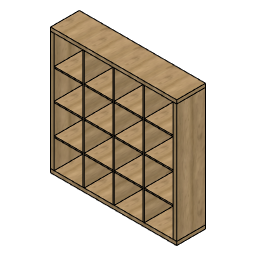
Kast+parametrisch+v5 (Autodesk Fusion 360 design; units mm, degrees)
part number: 123
Autodesk Fusion 360 part; units mm, degrees
sketch "Sketch1" plane through (0, 0, 0) normal (0, 0, 1) x (1, 0, 0)
  line L0 (0, 0) -> (50, 0)
  line L1 (50, 0) -> (50, 1654)
  line L2 (50, 1654) -> (0, 1654)
  line L3 (0, 1654) -> (0, 0)
  line L4 (0, 0) -> (1754, 0)
  line L5 (1754, 0) -> (1754, -50)
  line L6 (1754, -50) -> (0, -50)
  line L7 (0, -50) -> (0, 0)
  line L8 (450, 0) -> (468, 0)
  line L9 (468, 0) -> (468, 1654)
  line L10 (468, 1654) -> (450, 1654)
  line L11 (450, 1654) -> (450, 0)
  line L12 (50, 400) -> (450, 400)
  line L13 (450, 400) -> (450, 418)
  line L14 (450, 418) -> (50, 418)
  line L15 (50, 418) -> (50, 400)
  dimension "d7" = 1654
  dimension "d8" = 50
  dimension "d9" = 1754
  dimension "d10" = 50
  dimension "d12" = 18
  dimension "d13" = 400
  dimension "d14" = 1654
  dimension "d15" = 18
  dimension "d16" = 400
  constraint horizontal L0
  constraint vertical L1
  constraint horizontal L2
  constraint vertical L3
  constraint coincident L0.start L3.end
  constraint horizontal L4
  constraint vertical L5
  constraint horizontal L6
  constraint vertical L7
  constraint horizontal L8
  constraint vertical L9
  constraint horizontal L10
  constraint vertical L11
  constraint coincident L4 L8.start
  constraint horizontal L12
  constraint vertical L13
  constraint horizontal L14
  constraint vertical L15
  constraint coincident L11 L13.end
  constraint coincident L1 L12.start
  measures "d7" vertical distance of L0.start L2.end
  measures "d8" horizontal distance of L0.start L0.end
  measures "d9" horizontal distance of L5.end L6.end
  measures "d10" distance of L4 L6
  measures "d12" horizontal distance of L9.end L10.end
  measures "d13" distance of L1 L11
  measures "d14" vertical distance of L8.start L10.end
  measures "d15" distance of L12 L14
  measures "d16" distance of L4 L12
extrude "Extrude1" add sketch "Sketch1" along normal blind 400 contours L0 L4 L5 L6 L7 L8 makes body 1 in component "Dik Horizontaal"
extrude "Extrude1'" add sketch "Sketch1" along normal blind 400 separate body contours L0 L1 L2 L3 L4 L15 makes body 2 in component "Dik Vertikaal"
extrude "Extrude1''" add sketch "Sketch1" along normal blind 400 separate body contours L1 L11 L12 L13 L14 L15 makes body 3 in component "Dun Horizontaal"
extrude "Extrude1'''" add sketch "Sketch1" along normal blind 400 separate body contours L4 L8 L9 L10 L11 L13 makes body 4 in component "Dun Vertikaal"
pattern_linear "Patroon planken dun horizontaal" [suppressed]
pattern_linear "Patroon planken dun vertikaal" [suppressed]
pattern_linear "Patroon planken dik vertikaal" [suppressed]
pattern_linear "Patroon planken dik horizontaal" [suppressed]
component "Dik Horizontaal" placed x (1, 0, 0) y (0, 1, 0) z (0, 0, 1) at (0, 0, 0)
component "Dik Vertikaal" placed x (1, 0, 0) y (0, 1, 0) z (0, 0, 1) at (0, 0, 0)
component "Dun Horizontaal" placed x (1, 0, 0) y (0, 1, 0) z (0, 0, 1) at (0, 0, 0)
component "Dun Vertikaal" placed x (1, 0, 0) y (0, 1, 0) z (0, 0, 1) at (0, 0, 0)
component "Dun Vertikaal" placed x (1, 0, 0) y (0, 1, 0) z (0, 0, 1) at (418, 0, 0)
component "Dun Vertikaal" placed x (1, 0, 0) y (0, 1, 0) z (0, 0, 1) at (836, 0, 0)
component "Dik Vertikaal" placed x (1, 0, 0) y (0, 1, 0) z (0, 0, 1) at (1704, 0, 0)
component "Dun Horizontaal" placed x (1, 0, 0) y (0, 1, 0) z (0, 0, 1) at (0, 418, 0)
component "Dun Horizontaal" placed x (1, 0, 0) y (0, 1, 0) z (0, 0, 1) at (0, 836, 0)
component "Dun Horizontaal" placed x (1, 0, 0) y (0, 1, 0) z (0, 0, 1) at (418, 0, 0)
component "Dun Horizontaal" placed x (1, 0, 0) y (0, 1, 0) z (0, 0, 1) at (418, 418, 0)
component "Dun Horizontaal" placed x (1, 0, 0) y (0, 1, 0) z (0, 0, 1) at (418, 836, 0)
component "Dun Horizontaal" placed x (1, 0, 0) y (0, 1, 0) z (0, 0, 1) at (836, 0, 0)
component "Dun Horizontaal" placed x (1, 0, 0) y (0, 1, 0) z (0, 0, 1) at (836, 418, 0)
component "Dun Horizontaal" placed x (1, 0, 0) y (0, 1, 0) z (0, 0, 1) at (836, 836, 0)
component "Dun Horizontaal" placed x (1, 0, 0) y (0, 1, 0) z (0, 0, 1) at (1254, 0, 0)
component "Dun Horizontaal" placed x (1, 0, 0) y (0, 1, 0) z (0, 0, 1) at (1254, 418, 0)
component "Dun Horizontaal" placed x (1, 0, 0) y (0, 1, 0) z (0, 0, 1) at (1254, 836, 0)
component "Dik Horizontaal" placed x (1, 0, 0) y (0, 1, 0) z (0, 0, 1) at (0, 1704, 0)
equation "VakHoogte = 400 mm"
equation "VakBreedte = 400 mm"
equation "VakDiepte = 400 mm"
equation "AantalVertikaal = 4"
equation "AantalHorizontaal = 4"
equation "PlankDikteZei = 50 mm"
equation "d7 = ( AantalVertikaal * VakHoogte ) + ( ( AantalVertikaal - 1 ) * PlankDikteMid )"
equation "d8 = PlankDikteZei"
equation "d9 = ( VakBreedte * AantalHorizontaal ) + ( ( AantalHorizontaal - 1 ) * PlankDikteMid ) + ( PlankDikteZei * 2 )"
equation "d10 = PlankDikteZei"
equation "PlankDikteMid = 18 mm"
equation "d12 = PlankDikteMid"
equation "d13 = VakBreedte"
equation "d14 = ( AantalVertikaal * VakHoogte ) + ( ( AantalVertikaal - 1 ) * PlankDikteMid )"
equation "d15 = PlankDikteMid"
equation "d16 = VakHoogte"
equation "d17 = VakDiepte"
equation "d19 = VakDiepte"
equation "d21 = VakDiepte"
equation "d23 = VakDiepte"
equation "d25 = AantalVertikaal - 1"
equation "d26 = AantalHorizontaal"
equation "d27 = ( VakHoogte * -1 ) - PlankDikteMid"
equation "d28 = VakBreedte + PlankDikteMid"
equation "d29 = AantalHorizontaal - 1"
equation "d31 = VakBreedte + PlankDikteMid"
equation "d35 = ( VakBreedte * AantalHorizontaal ) + ( ( AantalHorizontaal - 1 ) * PlankDikteMid ) + PlankDikteZei"
equation "d39 = ( VakHoogte * AantalVertikaal ) + ( ( AantalVertikaal - 1 ) * PlankDikteMid ) + PlankDikteZei"
